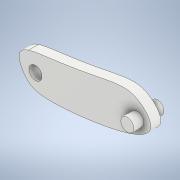
# Autodesk Inventor part: Component19
Saved by Autodesk Inventor 2022 (Build 260153000, 153)
## iProperties
Created: 2022-01-29
Part Number: Component19
Material: Generic
Document SubType Name: Modeling
Designer: Administrator
Density: 1 g/cm^3
Appearance: Default
Title: Component19
Author: Administrator
Autodesk Inventor part; units mm, degrees
ref_plane "YZ Plane" through (0, 0, 0) normal (1, 0, 0) x (0, 1, 0)
ref_plane "XZ Plane" through (0, 0, 0) normal (0, 1, 0) x (-1, 0, 0)
ref_plane "XY Plane" through (0, 0, 0) normal (0, 0, 1) x (1, 0, 0)
sketch "Sketch2" plane through (0, 0, 0) normal (0, 0, 1) x (1, 0, 0)
  circle A0 centre (27.9622, 4.8014) radius 3.25
  circle A1 centre (-22.8001, -0.7341) radius 3.25
  spline S0 degree 5 poles (-26.303, 7.2922) (-24.9205, 7.7366) (-21.689, 8.4515) (-15.6774, 9.1503) (-6.9174, 10.3062) (3.7458, 12.1452) (12.8293, 14.0988) (19.9856, 15.2853) (25.3324, 14.9647) (29.4316, 12.7518) (33.2982, 9.2808) (35.5102, 5.1998) (34.0987, 1.1236) (27.9236, -2.5003) (17.7665, -5.4503) (5.4371, -7.6312) (-6.8224, -8.9727) (-16.8971, -9.3866) (-23.6955, -8.5705) (-27.1603, -6.1813) (-30.6429, -1.0411) (-31.7962, 3.5227) (-29.9838, 5.7853) (-27.6854, 6.8478) (-26.303, 7.2922) knots 0 0 0 0 0 0 0.05 0.1 0.15 0.2 0.25 0.3 0.35 0.4 0.45 0.5 0.55 0.6 0.65 0.7 0.75 0.8 0.85 0.9 0.95 1 1 1 1 1 1 weights 1 1 1 1 1 1 1 1 1 1 1 1 1 1 1 1 1 1 1 1 1 1 1 1 1
  point P0 (0, 0)
  dimension "d6" = 6.5
  constraints: 2 centre point, 1 equal radius, 1 other
  measures "d6" diameter of A1
extrude "Extrusion1" add sketch "Sketch2" along normal blind 5 contours A0 | S0
extrude "Extrusion2" add sketch "Sketch2" against normal blind 5 contours A0
sketch "Sketch3" plane through (0, 0, 5) normal (0, 0, 1) x (1, 0, 0)
  circle A0 centre (27.9622, 4.8014) radius 3.25 projected
  circle A1 centre (-22.8001, -0.7341) radius 3.25 projected
  point P0 (0, 0)
  point P1 (-26.303, 7.2922)
  constraints: 1 other
extrude "Extrusion3" add sketch "Sketch3" along normal blind 5 contours A0
equation "\"d6\" = R"
equation "\"d0\" = thickness"
equation "\"d2\" = thickness"
equation "\"d4\" = thickness"
equation "\"R\" = 6.5"
equation "\"thickness\" = 5"
equation "\"width\" = 6.5"
equation "\"R1\" = 9"
body "Solid1"
